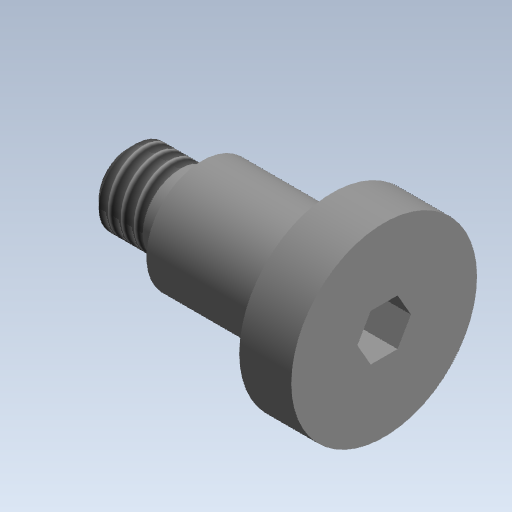
# Autodesk Inventor part: DBS4-7-4
Saved by Autodesk Inventor 2020 (Build 240168000, 168)
## iProperties
Part Number: DBS4-7-4
Material: 一般
Description: 既製品
Vendor: MISUMI
Document SubType Name: Modeling
Designer: partserver
Manufacturer: MISUMI
Mass: 0.452309 g
Surface Area: 4.46265 cm^2
Volume: 0.452309 cm^3
Density: 1 g/cm^3
Appearance: PSOLRGB-175-175-175
Category: PARTsolutions
Company: MISUMI
PSOL_IDENT_0: {$CADENAS_DATA\23d-libs\misumi\metric\27_screws_nuts\dbb.prj},176 {VTYP=3D},{NB=DBS4-7-4},{LINA=DBS4
PSOL_IDENT_1: -7-4},{NN=DBB, DBM, DBS},{DATE=30.06.2021 13:09:28},{GEOMDATE=15.01.2020 08:58:15},{VERSION=},{LINEI
PSOL_IDENT_2: D=20},{WBVAR=MAT,ST,L,F},{WBNUMERIC=L,F}  {NB=DBS4-7-4},{LINA=DBS4-7-4},{KT=DUMMY},{PN=DBS4-7-4},{TY
PSOL_IDENT_3: PE=DB},{MAT=S},{ST=-},{STALG= '-','-'},{M=4},{L=7},{LALG=3,4,5,6,7,8,10},{F=4},{FALG=4,5,6,8},{E=2.8
PSOL_IDENT_4: },{DHH7=6},{A=10},{B=2.5},{LL=1.2},{HH1=2.5}
NB: DBS4-7-4
NN: DBB, DBM, DBS
NT: Stepped Screws - Low Head Selectable
NBSYN: $PN.
LINA: DBS4-7-4
CATALOG: Misumi
PN: DBS4-7-4
TYPE: DB
MAT: 303 Stainless Steel
ST: -
M: 4
L: 7
F: 4
E: 2.8
DHH7: 6
A: 10
B: 2.5
LL: 1.2
HH1: 2.5
SUPPLIER: MISUMI
ARTICLENO: DBS4-7-4
BOMINFO: DBS4-7-4
CREATOR: CADENAS GmbH
Title: DBS4-7-4
Author: Cadenas PARTsolutions
Autodesk Inventor part; units mm, degrees
ref_plane "YZ Plane" through (0, 0, 0) normal (1, 0, 0) x (0, 1, 0)
ref_plane "XZ Plane" through (0, 0, 0) normal (0, 1, 0) x (-1, 0, 0)
ref_plane "XY Plane" through (0, 0, 0) normal (0, 0, 1) x (1, 0, 0)
sketch "Sketch_1" plane through (0, 0, 0) normal (0, 0, 1) x (1, 0, 0)
  line L0 (4, 0) -> (-9.8, 0)
  line L1 (-9.8, 0) -> (-9.8, 5)
  line L2 (-9.8, 5) -> (-7, 5)
  line L3 (-7, 5) -> (-7, 3)
  line L4 (-7, 3) -> (0, 3)
  line L5 (0, 3) -> (0, 2)
  line L6 (0, 2) -> (3.5705, 2)
  line L7 (3.5705, 2) -> (4, 1.5705)
  line L8 (4, 1.5705) -> (4, 0)
  line L9 (4, 0) -> (-9.8, 0)
  constraints: 20 end point
revolve "Revolution1" add sketch "Sketch_1" angle 360 about axis through (4, 0, 0) along (1, 0, 0)
thread "Thread1" size "M4x0.7" class "6g" standard "ISO Metric profile" length 2.3705
sketch "Sketch_2" plane through (-9.8, 0, 0) normal (-1, 0, 0) x (0, 1, 0)
  line L0 (-1.4434, 0) -> (-0.7217, -1.25)
  line L1 (-0.7217, -1.25) -> (0.7217, -1.25)
  line L2 (0.7217, -1.25) -> (1.4434, 0)
  line L3 (1.4434, 0) -> (0.7217, 1.25)
  line L4 (0.7217, 1.25) -> (-0.7217, 1.25)
  line L5 (-0.7217, 1.25) -> (-1.4434, 0)
  constraints: 12 end point
extrude "Extrusion1" cut sketch "Sketch_2" against normal blind 2.5
sketch "Sketch_3" plane through (0, 0, 0) normal (0, 0, 1) x (1, 0, 0)
  line L0 (-6.5783, 0) -> (-7.3, 0)
  line L1 (-7.3, 0) -> (-7.3, 1.25)
  line L2 (-7.3, 1.25) -> (-6.5783, 0)
  line L3 (-6.5783, 0) -> (-7.3, 0)
  constraints: 8 end point
revolve "Revolution2" cut sketch "Sketch_3" angle 360 about axis through (-6.5783, 0, 0) along (1, 0, 0)
body "Solid1"
